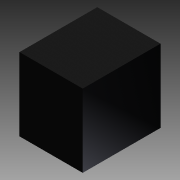
# Autodesk Inventor part: battery model
Saved by Autodesk Inventor 2012 (Build 160160000, 160)
## iProperties
Created: 2011-10-05
Part Number: battery model
Material: Default
Document SubType Name: Modeling
Designer: Antonella
Density: 1 g/cm^3
Author: Antonella
Autodesk Inventor part; units mm, degrees
ref_plane "YZ Plane" through (0, 0, 0) normal (1, 0, 0) x (0, 1, 0)
ref_plane "XZ Plane" through (0, 0, 0) normal (0, 1, 0) x (-1, 0, 0)
ref_plane "XY Plane" through (0, 0, 0) normal (0, 0, 1) x (1, 0, 0)
sketch "Sketch1" plane through (0, 0, 0) normal (0, 0, 1) x (1, 0, 0)
  line L0 (-21.8487, 16.7227) -> (143.2513, 16.7227)
  line L1 (143.2513, 16.7227) -> (143.2513, -173.7773)
  line L2 (143.2513, -173.7773) -> (-21.8487, -173.7773)
  line L3 (-21.8487, -173.7773) -> (-21.8487, 16.7227)
  point P0 (0, 0)
  dimension "d0" = 165.1
  dimension "d1" = 190.5
  constraints: 8 end point, 2 parallel, 1 horizontal, 1 perpendicular
  measures "d0" distance of L0.start L0.end
  measures "d1" distance of L2.end L0.start
extrude "Extrusion1" add sketch "Sketch1" along normal blind 203.2
body "Solid1"
